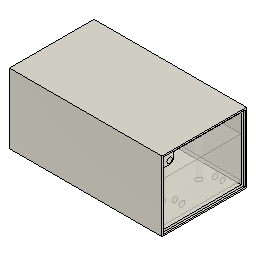
Juicebox (Autodesk Fusion 360 design; units mm, degrees)
Autodesk Fusion 360 part; units mm, degrees
sketch "footprint" plane through (0, 0, 0) normal (0, 0, 1) x (1, 0, 0) in component "IP5328P"
  line L0 (0, 0) -> (65, 0)
  line L1 (65, 0) -> (65, 32.5)
  line L2 (65, 32.5) -> (0, 32.5)
  line L3 (0, 32.5) -> (0, 0)
  line L4 (32.5, 32.5) -> (32.5, 0) construction
  line L5 (65, 16.25) -> (0, 16.25) construction
  line L6 (62.5, 29.75) -> (2.5, 29.75) construction
  line L7 (2.5, 29.75) -> (2.5, 2.75) construction
  line L8 (2.5, 2.75) -> (62.5, 2.75) construction
  line L9 (62.5, 2.75) -> (62.5, 29.75) construction
  line L10 (62.5, 29.75) -> (2.5, 2.75) construction
  line L11 (2.5, 29.75) -> (62.5, 2.75) construction
  circle A0 centre (62.5, 29.75) radius 1.5
  circle A1 centre (62.5, 2.75) radius 1.5
  circle A2 centre (2.5, 2.75) radius 1.5
  circle A3 centre (2.5, 29.75) radius 1.5
  line L12 (8, 32.5) -> (21, 32.5)
  line L13 (21, 32.5) -> (21, 21.5)
  line L14 (21, 21.5) -> (8, 21.5)
  line L15 (8, 21.5) -> (8, 32.5)
  line L16 (28, 32.5) -> (37, 32.5)
  line L17 (37, 32.5) -> (37, 25.5)
  line L18 (37, 25.5) -> (28, 25.5)
  line L19 (28, 25.5) -> (28, 32.5)
  line L20 (44, 32.5) -> (57, 32.5)
  line L21 (57, 32.5) -> (57, 21.5)
  line L22 (57, 21.5) -> (44, 21.5)
  line L23 (44, 21.5) -> (44, 32.5)
  line L24 (0, 7) -> (7, 7)
  line L25 (7, 7) -> (7, 15)
  line L26 (7, 15) -> (0, 15)
  line L27 (0, 15) -> (0, 7)
  line L28 (0, 21) -> (4, 21)
  line L29 (4, 21) -> (4, 26)
  line L30 (4, 26) -> (0, 26)
  line L31 (0, 26) -> (0, 21)
  line L32 (1, 21) -> (1, 26)
  point P0 (32.5, 16.25)
  dimension "d1" = 65
  dimension "d2" = 32.5
  dimension "d5" = 60
  dimension "d6" = 27
  dimension "d7" = 3
  dimension "d8" = 3
  dimension "d9" = 3
  dimension "d10" = 3
  dimension "d11" = 13
  dimension "d12" = 11
  dimension "d13" = 8
  dimension "d14" = 9
  dimension "d15" = 7
  dimension "d16" = 7
  dimension "d17" = 8
  dimension "d27" = 7
  dimension "d28" = 8
  dimension "d29" = 7
  dimension "d30" = 4
  dimension "d31" = 5
  dimension "d32" = 6
  dimension "d179" = 3
  constraint horizontal L0
  constraint vertical L1
  constraint horizontal L2
  constraint vertical L3
  constraint coincident L0.start L3.end
  constraint midpoint L2 L4.start
  constraint perpendicular L2 L4
  constraint midpoint L1 L5.start
  constraint midpoint L3 L5.end
  constraint horizontal L6
  constraint perpendicular L6 L7
  constraint parallel L6 L8
  constraint parallel L7 L9
  constraint coincident L10 P0
  constraint coincident L11 P0
  constraint midpoint L5 P0
  constraint coincident L6.start L9.end
  constraint coincident L8.end L9.start
  constraint coincident L7.end L8.start
  constraint coincident L6.end L7.start
  constraint horizontal L12
  constraint vertical L13
  constraint horizontal L14
  constraint vertical L15
  constraint coincident L2 L12.start
  constraint horizontal L16
  constraint vertical L17
  constraint horizontal L18
  constraint vertical L19
  constraint coincident L2 L16.start
  constraint horizontal L20
  constraint vertical L21
  constraint horizontal L22
  constraint vertical L23
  constraint coincident L2 L20.start
  constraint equal L14 L22
  constraint equal L13 L23
  constraint horizontal L24
  constraint vertical L25
  constraint horizontal L26
  constraint vertical L27
  constraint coincident L3 L24.start
  constraint horizontal L28
  constraint vertical L29
  constraint horizontal L30
  constraint vertical L31
  constraint coincident L3 L28.start
  constraint coincident L28 L32.start
  constraint coincident L30 L32.end
  constraint perpendicular L30 L32
  measures "d1" distance of L0.start L0.end
  measures "d2" distance of L0.start L2.end
  measures "d5" distance of L7.end L8.end
  measures "d6" distance of L6.end L7.end
  measures "d7" diameter of A0
  measures "d8" diameter of A1
  measures "d9" diameter of A2
  measures "d10" diameter of A3
  measures "d11" distance of L12.start L12.end
  measures "d12" distance of L12.start L14.end
  measures "d13" distance of L3 L15
  measures "d14" distance of L16.start L16.end
  measures "d15" distance of L16.start L18.end
  measures "d16" distance of L13 L19
  measures "d17" distance of L1 L21
  measures "d27" distance of L24.start L24.end
  measures "d28" distance of L24.start L26.end
  measures "d29" distance of L0 L24
  measures "d30" distance of L28.start L28.end
  measures "d31" distance of L28.start L30.end
  measures "d32" distance of L26 L28
  measures "d179" distance of L29 L32
extrude "Extrude1" add sketch "footprint" along normal blind 1.6 contours L0 L1 L2 L3 L13 L14 L15 L17 L18 L19 L21 L22 L23 L24 L25 L26 L28 L29 L30 | L3 L24 L25 L26 L27 | L3 L28 L30 L31 L32 | L28 L29 L30 L32 | L2 L16 L17 L18 L19 makes body 1 in component "IP5328P"
extrude "Extrude2" add sketch "footprint" along normal blind 6 separate body contours L2 L20 L21 L22 L23 | L2 L12 L13 L14 L15 makes body 2 at (12.3333, 28.8333, 0) makes body 3 at (48.3333, 28.8333, 0) in component "IP5328P"
extrude "Extrude3" add sketch "footprint" along normal blind 4 from surface at 1.6 separate body contours L2 L16 L17 L18 L19 makes body 4 in component "IP5328P"
sketch "ports_front" plane through (0, 32.5, 0) normal (0, 1, 0) x (-1, 0, 0) in component "IP5328P"
  line L0 (-57, 0) -> (-44, 0)
  line L1 (-44, 0) -> (-44, 6)
  line L2 (-44, 6) -> (-57, 6)
  line L3 (-57, 6) -> (-57, 0)
  line L4 (-21, 0) -> (-8, 0)
  line L5 (-8, 0) -> (-8, 6)
  line L6 (-8, 6) -> (-21, 6)
  line L7 (-21, 6) -> (-21, 0)
  line L8 (-37, 1.6) -> (-28, 1.6)
  line L9 (-28, 1.6) -> (-28, 5.6)
  line L10 (-28, 5.6) -> (-37, 5.6)
  line L11 (-37, 5.6) -> (-37, 1.6)
  line L12 (-35, 1.6) -> (-30, 1.6)
  arc A0 (-30, 1.6) -> (-30, 5.6) centre (-30, 3.6) ccw
  line L13 (-30, 5.6) -> (-35, 5.6)
  arc A1 (-35, 5.6) -> (-35, 1.6) centre (-35, 3.6) ccw
  line L14 (-37, 3.6) -> (-28, 3.6) construction
  constraint tangent L12 A0
  constraint tangent A0 L13
  constraint parallel L12 L13
  constraint tangent L13 A1
  constraint tangent L12 A1
  constraint midpoint A1 L14.start
  constraint midpoint A0 L14.end
  constraint midpoint L9 L14.end
  constraint perpendicular L9 L14
  constraint midpoint L11 L14.start
  constraint collinear L10 L13
extrude "Extrude4" cut sketch "ports_front" against normal up to surface (7 mm away) contours L8 L10 L12 A0 L13 A1 keep common part bodies 4 in component "IP5328P"
extrude "Extrude5" add sketch "footprint" along normal blind 3 from surface at 1.6 separate body contours L3 L24 L25 L26 L27 makes body 5 in component "IP5328P"
extrude "Extrude6" add sketch "footprint" along normal blind 3.2 from surface at 1.6 separate body contours L3 L28 L30 L31 L32 | L28 L29 L30 L32 makes body 6 in component "IP5328P"
sketch "ports_side" plane through (0, 0, 0) normal (-1, 0, 0) x (0, -1, 0) in component "IP5328P"
  line L0 (-26, 1.6) -> (-21, 1.6)
  line L1 (-21, 1.6) -> (-21, 4.8)
  line L2 (-21, 4.8) -> (-26, 4.8)
  line L3 (-26, 4.8) -> (-26, 1.6)
  circle A0 centre (-23.5, 3.2) radius 1
  line L4 (-26, 3.2) -> (-21, 3.2) construction
  line L5 (-23.5, 4.8) -> (-23.5, 1.6) construction
  line L6 (-15, 1.6) -> (-7, 1.6)
  line L7 (-7, 1.6) -> (-7, 4.6)
  line L8 (-7, 4.6) -> (-15, 4.6)
  line L9 (-15, 4.6) -> (-15, 1.6)
  line L10 (-15, 4.6) -> (-7, 4.6)
  line L11 (-15, 4.6) -> (-15, 3.4)
  line L12 (-13, 1.6) -> (-9, 1.6)
  line L13 (-13, 1.6) -> (-15, 3.4)
  line L14 (-7, 4.6) -> (-7, 3.4)
  line L15 (-15, 4.6) -> (-15, 3.4)
  line L16 (-7, 3.4) -> (-9, 1.6)
  dimension "d39" = 2
  dimension "d42" = 1.2
  dimension "d43" = 4
  constraint midpoint L3 L4.start
  constraint midpoint L1 L4.end
  constraint midpoint L2 L5.start
  constraint midpoint L0 L5.end
  constraint midpoint A0.centre L4
  constraint coincident L8 L9.start
  constraint coincident L7.end L8.start
  constraint perpendicular L7 L10
  constraint coincident L8.end L9.start
  constraint perpendicular L10 L11
  constraint coincident L6 L12.start
  constraint perpendicular L9 L12
  constraint midpoint L6 L12
  constraint coincident L7 L14.end
  constraint equal L14 L15
  measures "d39" diameter of A0
  measures "d42" distance of L8.end L11.end
  measures "d43" distance of L12.start L12.end
extrude "Extrude7" cut sketch "ports_side" against normal blind 1 contours L0 L1 L2 L3 bodies 6 in component "IP5328P"
extrude "Extrude8" cut sketch "ports_side" against normal blind 7 contours L6 L7 L8 L9 L10 L11 L12 L13 L14 L15 L16 keep common part bodies 5 in component "IP5328P"
sketch "Bottom_Screws" plane through (0, 0, 0) normal (0, 0, 1) x (1, 0, 0) in component "Battery_Holder"
  line L0 (0, -9.5) -> (80, -9.5)
  line L1 (80, -9.5) -> (80, 32.5)
  line L2 (80, 32.5) -> (0, 32.5)
  line L3 (0, 32.5) -> (0, -9.5)
  line L4 (40, -9.5) -> (40, 32.5) construction
  line L5 (80, 11.5) -> (0, 11.5) construction
  line L6 (12, 1.5) -> (68, 1.5) construction
  line L7 (68, 1.5) -> (68, 21.5) construction
  line L8 (68, 21.5) -> (12, 21.5) construction
  line L9 (12, 21.5) -> (12, 1.5) construction
  line L10 (12, 1.5) -> (68, 21.5) construction
  line L11 (68, 1.5) -> (12, 21.5) construction
  circle A0 centre (68, 1.5) radius 1.5
  circle A1 centre (12, 1.5) radius 1.5
  circle A2 centre (12, 21.5) radius 1.5
  circle A3 centre (68, 21.5) radius 1.5
  line L12 (0, 0) -> (65, 0)
  line L13 (65, 0) -> (65, 32.5)
  line L14 (0, 32.5) -> (0, 0)
  line L15 (65, 32.5) -> (0, 32.5)
  point P0 (40, 11.5)
  point P1 (0, 32.5)
  dimension "d46" = 80
  dimension "d47" = 42
  dimension "d48" = 56
  dimension "d49" = 20
  dimension "d50" = 3
  dimension "d51" = 3
  dimension "d52" = 3
  dimension "d53" = 3
  constraint horizontal L0
  constraint vertical L1
  constraint horizontal L2
  constraint vertical L3
  constraint midpoint L0 L4.start
  constraint midpoint L2 L4.end
  constraint midpoint L1 L5.start
  constraint midpoint L3 L5.end
  constraint horizontal L6
  constraint perpendicular L6 L7
  constraint parallel L6 L8
  constraint parallel L7 L9
  constraint coincident L10 P0
  constraint coincident L11 P0
  constraint midpoint L5 P0
  constraint coincident L6.end L7.start
  constraint coincident L6.start L9.end
  constraint coincident L8.end L9.start
  constraint coincident L7.end L8.start
  constraint coincident P1 L2.end
  measures "d46" distance of L0.start L0.end
  measures "d47" distance of L0.start L2.end
  measures "d48" distance of L7.end L8.end
  measures "d49" distance of L6.end L7.end
  measures "d50" diameter of A0
  measures "d51" diameter of A1
  measures "d52" diameter of A2
  measures "d53" diameter of A3
extrude "Extrude1'" add sketch "Bottom_Screws" against normal blind 22 from surface at -2 separate body makes body 7 in component "Battery_Holder"
sketch "Side_screws" plane through (80, 0, 0) normal (1, 0, 0) x (0, 1, 0) in component "Battery_Holder"
  line L0 (32.5, -2) -> (-9.5, -2)
  line L1 (-9.5, -2) -> (-9.5, -24)
  line L2 (-9.5, -24) -> (32.5, -24)
  line L3 (32.5, -24) -> (32.5, -2)
  line L4 (22.5, -24) -> (22.5, -19) construction
  line L5 (32.5, -19) -> (22.5, -19) construction
  line L6 (11.5, -2) -> (11.5, -24)
  circle A0 centre (22.5, -19) radius 1.25
  circle A1 centre (0.5, -19) radius 1.25
  line L7 (-9.5, -19) -> (0.5, -19) construction
  line L8 (0.5, -24) -> (0.5, -19) construction
  dimension "d152" = 5
  dimension "d153" = 10
  dimension "d154" = 2.5
  constraint coincident L2 L4.start
  constraint vertical L4
  constraint coincident L3 L5.start
  constraint horizontal L5
  constraint midpoint L0 L6.start
  constraint midpoint L2 L6.end
  constraint coincident L4.end L5.end
  constraint symmetric L4.start L6 L8.start
  constraint symmetric L4.end L6 A1.centre
  constraint symmetric L5.start L6 L7.start
  constraint symmetric L6 A0 A1
  measures "d152" distance of L4.start L4.end
  measures "d153" distance of L4.end L5.start
  measures "d154" diameter of A0
sketch "Shell_frame" plane through (80, 0, 0) normal (1, 0, 0) x (0, 1, 0) in component "Enclosure"
  line L0 (32.5, -2) -> (-9.5, -2)
  line L1 (-9.5, -2) -> (-9.5, -24)
  line L2 (-9.5, -24) -> (32.5, -24)
  line L3 (32.5, -24) -> (32.5, -2)
  line L4 (21.5, 0) -> (32.5, 0)
  line L5 (32.5, 0) -> (32.5, 6)
  line L6 (32.5, 6) -> (21.5, 6)
  line L7 (21.5, 6) -> (21.5, 0)
  line L8 (-11.5, 10) -> (34.5, 10)
  line L9 (34.5, 10) -> (34.5, -28)
  line L10 (34.5, -28) -> (-11.5, -28)
  line L11 (-11.5, -28) -> (-11.5, 10)
  line L12 (-9.5, -26) -> (32.5, -26)
  line L13 (32.5, -26) -> (32.5, 8)
  line L14 (32.5, 8) -> (-9.5, 8)
  line L15 (-9.5, 8) -> (-9.5, -26)
  line L16 (-10.3, 8.8) -> (33.3, 8.8)
  line L17 (33.3, 8.8) -> (33.3, -26.8)
  line L18 (33.3, -26.8) -> (-10.3, -26.8)
  line L19 (-10.3, -26.8) -> (-10.3, 8.8)
  line L20 (-10.7, 9.2) -> (33.7, 9.2)
  line L21 (33.7, 9.2) -> (33.7, -27.2)
  line L22 (33.7, -27.2) -> (-10.7, -27.2)
  line L23 (-10.7, -27.2) -> (-10.7, 9.2)
  line L24 (-4.3682, 9.2) -> (-4.3682, 5)
  line L25 (-6.3682, 3) -> (-10.7, 3)
  arc A0 (-6.3682, 3) -> (-4.3682, 5) centre (-6.3682, 5) ccw
  circle A1 centre (-6.3682, 5) radius 1.25
  dimension "d129" = 2
  dimension "d130" = 2
  dimension "d131" = 4
  dimension "d132" = 4
  dimension "d133" = 2
  dimension "d134" = 2
  dimension "d135" = 1.2
  dimension "d136" = 0.8
  dimension "d155" = 2
  dimension "d156" = 2.5
  constraint horizontal L8
  constraint vertical L9
  constraint horizontal L10
  constraint vertical L11
  constraint horizontal L12
  constraint vertical L13
  constraint horizontal L14
  constraint vertical L15
  constraint collinear L1 L15
  constraint collinear L3 L13
  constraint coincident L20 L24.start
  constraint perpendicular L14 L24
  constraint coincident L23 L25.end
  constraint perpendicular L23 L25
  constraint tangent L24 A0
  constraint tangent L25 A0
  constraint concentric A0 A1
  measures "d129" distance of L1 L11
  measures "d130" distance of L3 L9
  measures "d131" distance of L6 L8
  measures "d132" distance of L2 L10
  measures "d133" distance of L8 L14
  measures "d134" distance of L10 L12
  measures "d155" radius of A0
  measures "d156" diameter of A1
extrude "Extrude12" add sketch "Shell_frame" against normal up to surface (80 mm away) separate body contours L1 L3 L5 L12 L13 L14 L15 L16 L17 L18 L19 L24 L25 | L14 L15 L16 L19 L24 L25 | L16 L19 L20 L23 L24 L25 | L16 L17 L18 L19 L20 L21 L22 L23 L24 L25 | L8 L9 L10 L11 makes body 8 in component "Enclosure"
extrude "Extrude13" add sketch "Shell_frame" against normal blind 2 from surface at -80 contours L0 L1 L2 L3 L13 L15 | L1 L3 L5 L12 L13 L14 L15 L16 L17 L18 L19 L24 L25 | L0 L4 L6 L7 L13 L14 L15 L24 L25 A0 | L2 L12 L13 L15 | L4 L5 L6 L7 L13 | L14 L15 L16 L19 L24 L25 | L14 L15 L24 L25 A0 | L16 L19 L20 L23 L24 L25 | L16 L17 L18 L19 L20 L21 L22 L23 L24 L25 | L8 L9 L10 L11 | A1 bodies 8 in component "Enclosure"
extrude "Extrude14" cut sketch "ports_front" along normal up to surface (2 mm away) contours L0 L1 L2 L3 | L4 L5 L6 L7 | L8 L10 L12 A0 L13 A1 bodies 8 in component "Enclosure"
extrude "Extrude19" add sketch "Shell_frame" against normal blind 2 contours L14 L15 L24 L25 A0 bodies 8 in component "Enclosure"
extrude "Extrude15" cut sketch "ports_side" along normal up to surface (2 mm away) contours L0 L1 L2 L3 | A0 | L6 L7 L8 L9 L10 L11 L12 L13 L14 L15 L16 bodies 8 in component "Enclosure"
extrude "Extrude16" add sketch "Shell_frame" along normal blind 4 separate body contours L0 L1 L2 L3 L13 L15 | L1 L3 L5 L12 L13 L14 L15 L16 L17 L18 L19 L24 L25 | L0 L4 L6 L7 L13 L14 L15 L24 L25 A0 | L2 L12 L13 L15 | L4 L5 L6 L7 L13 | L14 L15 L16 L19 L24 L25 | L14 L15 L24 L25 A0 | L16 L19 L20 L23 L24 L25 | L16 L17 L18 L19 L20 L21 L22 L23 L24 L25 | L8 L9 L10 L11 | A1 makes body 9 in component "Enclosure"
extrude "Extrude18" cut sketch "Shell_frame" along normal blind 1.6 contours L16 L19 L20 L23 L24 L25 | L16 L17 L18 L19 L20 L21 L22 L23 L24 L25 | L8 L9 L10 L11 bodies 9 in component "Enclosure"
extrude "Extrude17" add sketch "Shell_frame" along normal blind 1 contours L8 L9 L10 L11 bodies 8 in component "Enclosure"
sketch "Screw_bores" plane through (84, 0, 0) normal (1, 0, 0) x (0, 1, 0) in component "Enclosure"
  line L0 (-11.5, -28) -> (34.5, -28)
  line L1 (34.5, -28) -> (34.5, 10)
  line L2 (34.5, 10) -> (-11.5, 10)
  line L3 (-11.5, 10) -> (-11.5, -28)
  circle A0 centre (-6.3682, 5) radius 1.25
  circle A1 centre (0.5, -19) radius 1.25
  circle A2 centre (22.5, -19) radius 1.25
hole "Hole2" at (84, -6.3682, 5) at (84, 0.5, -19) at (84, 22.5, -19) direction (-1, 0, 0) diameter 2.9 depth 8 tip angle 180 counterbore diameter 5.5 counterbore depth 2.5 bodies 7 in component "Battery_Holder"
hole "Hole2'" at (84, -6.3682, 5) at (84, 0.5, -19) at (84, 22.5, -19) direction (-1, 0, 0) diameter 2.9 depth 8 tip angle 180 counterbore diameter 5.5 counterbore depth 2.5 bodies 8 9 in component "Enclosure"
sketch "Screw_bores_back" plane through (-2, 0, 0) normal (-1, 0, 0) x (0, -1, 0) in component "Enclosure"
  line L0 (-9, 1.6) -> (-13, 1.6)
  line L1 (-13, 1.6) -> (-15, 3.4)
  line L2 (-15, 3.4) -> (-15, 4.6)
  line L3 (-15, 4.6) -> (-7, 4.6)
  line L4 (-7, 4.6) -> (-7, 3.4)
  line L5 (-7, 3.4) -> (-9, 1.6)
  line L6 (-21, 1.6) -> (-26, 1.6)
  line L7 (-26, 1.6) -> (-26, 4.8)
  line L8 (-26, 4.8) -> (-21, 4.8)
  line L9 (-21, 4.8) -> (-21, 1.6)
  line L10 (-34.5, 10) -> (-34.5, -28)
  line L11 (-34.5, -28) -> (11.5, -28)
  line L12 (11.5, -28) -> (11.5, 10)
  line L13 (11.5, 10) -> (-34.5, 10)
  circle A0 centre (-22.5, -19) radius 1.25
  circle A1 centre (-0.5, -19) radius 1.25
  circle A2 centre (-23.5, 3.2) radius 1
  line L14 (-21.4, 2) -> (-24.6465, 2)
  line L15 (-24.6465, 2) -> (-24.6465, 4.4)
  line L16 (-24.6465, 4.4) -> (-21.4, 4.4)
  line L17 (-21.4, 4.4) -> (-21.4, 2)
  line L18 (-24.6465, 3.9131) -> (-26, 3.9131)
  line L19 (-24.6465, 3.2) -> (-26, 3.2)
  line L20 (-24.6465, 2.4869) -> (-26, 2.4869)
  dimension "d180" = 0.4
  dimension "d181" = 0.4
  dimension "d182" = 0.4
  constraint horizontal L14
  constraint vertical L15
  constraint horizontal L16
  constraint vertical L17
  constraint coincident L15 L18.start
  constraint coincident L7 L18.end
  constraint perpendicular L7 L18
  constraint midpoint L15 L19.start
  constraint perpendicular L15 L19
  constraint symmetric L18.start L19 L20.start
  constraint symmetric L18.end L19 L20.end
  measures "d180" distance of L8 L16
  measures "d181" distance of L6 L14
  measures "d182" distance of L9 L17
hole "Hole3" at (-2, 22.5, -19) at (-2, 0.5, -19) direction (1, 0, 0) diameter 2.9 depth 8 tip angle 180 counterbore diameter 5.5 counterbore depth 2.5 bodies 7 in component "Battery_Holder"
hole "Hole3'" at (-2, 22.5, -19) at (-2, 0.5, -19) direction (1, 0, 0) diameter 2.9 depth 8 tip angle 180 counterbore diameter 5.5 counterbore depth 2.5 bodies 8 in component "Enclosure"
extrude "Extrude22" add sketch "Screw_bores_back" along normal blind 1 from surface at -2 contours L7 L15 L19 L20 | L7 L15 L18 L19 bodies 8 in component "Enclosure"
extrude "Extrude20" add sketch "Screw_bores_back" against normal up to surface (2 mm away) contours L14 L15 L16 L17 | A2 bodies 8 in component "Enclosure"
component "IP5328P" placed x (1, 0, 0) y (0, 1, 0) z (0, 0, 1) at (0, 0, 0)
component "Battery_Holder" placed x (1, 0, 0) y (0, 1, 0) z (0, 0, 1) at (0, 0, 0)
component "Enclosure" placed x (1, 0, 0) y (0, 1, 0) z (0, 0, 1) at (0, 0, 0)
hidden bodies 9
equation "d130 = d129"
equation "d131 = d129 + 2 mm"
equation "d132 = d129 + 2 mm"
equation "d133 = d129"
equation "d134 = d129"
named bodies: "PCB", "USBA_2", "USBA_1", "USBC", "microUSB", "Button", "Case_shell", "Case_cover"
